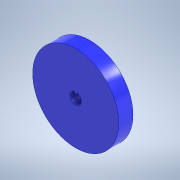
# Autodesk Inventor part: celestronMountDecHandle
Saved by Autodesk Inventor 2021.1 (Build 251245000, 245)
## iProperties
Created: 2020-07-29
Part Number: celestronMountDecHandle
Material: PC/ABS Plastic
Document SubType Name: Modeling
Designer: robst
Density: 0.357273 g/cm^3
Appearance: Blue - Wall Paint - Glossy
Author: robst
Autodesk Inventor part; units mm, degrees
ref_plane "YZ Plane" through (0, 0, 0) normal (1, 0, 0) x (0, 1, 0)
ref_plane "XY Plane" through (0, 0, 0) normal (0, 0, 1) x (1, 0, 0)
sketch "Sketch1" plane through (0, 0, 0) normal (0, 0, 1) x (1, 0, 0)
  circle A0 centre (0, 0) radius 38.1
  dimension "d0" = 76.2
  constraints: 1 centre point, 1 coincident
  measures "d0" diameter of A0
extrude "Extrusion1" add sketch "Sketch1" against normal blind 12.7
sketch "Sketch2" plane through (0, 0, -12.7) normal (0, 0, -1) x (-1, 0, 0)
  circle A0 centre (0, 0) radius 15.1765
  dimension "d3" = 30.353
  constraints: 1 centre point, 1 coincident
  measures "d3" diameter of A0
extrude "Extrusion2" add sketch "Sketch2" along normal blind 12.7
sketch "Sketch3" plane through (0, 0, 0) normal (0, 0, 1) x (1, 0, 0)
  arc A0 (-1.1906, 4.8732) -> (1.1906, 4.8732) centre (0, 0) ccw
  line L0 (-1.1906, 4.8732) -> (-1.1906, 3.4285)
  line L1 (-1.1906, 3.4285) -> (1.1906, 3.4285)
  line L2 (1.1906, 3.4285) -> (1.1906, 4.8732)
  circle A1 centre (0, 0) radius 15.1765 projected
  dimension "d6" = 10.033
  dimension "d7" = 2.3813
  dimension "d8" = 1.4446
  dimension "d15" = 10.16
  constraints: 6 end point, 2 point on circle, 2 vertical, 1 centre point, 1 coincident, 1 horizontal, 1 parallel
  measures "d6" diameter of A0
  measures "d7" distance of L0.end L1.end
  measures "d8" distance of L0.start L0.end
  measures "d15" radial gap between concentric circles of A0 A1
extrude "Extrusion3" cut sketch "Sketch3" against normal through all contours L0 L1 L2 A0
ref_plane "Work Plane2" through (0, -15.1765, 0) normal (0, 1, 0) x (-1, 0, 0)
sketch "Sketch4" plane through (0, -15.1765, 0) normal (0, 1, 0) x (-1, 0, 0)
  line L0 (-15.1765, -12.7) -> (-15.1765, -25.4) projected
  line L1 (15.1765, -12.7) -> (15.1765, -25.4) projected
  line L2 (-38.1, -12.7) -> (38.1, -12.7) projected
  line L3 (-15.1765, -25.4) -> (15.1765, -25.4) projected
  line L4 (0, -25.4) -> (0, -12.7) construction
  point P0 (0, 0)
  point P1 (0, -19.05)
  constraints: 3 midpoint, 2 end point
hole "Hole1" at (0, -15.1765, -19.05) direction (0, 1, 0) diameter 5.1054 depth 11.43 counterbore diameter 6.5278 counterbore depth 7.874 clearance for "Hex Machine Screw" size "#10" standard "Ansi Unified Screw Threads"
equation "\"d0\" = outerDiameter"
equation "\"d1\" = handleThickness"
equation "\"d3\" = shaftOutsideDiameter"
equation "\"d4\" = shaftLength"
equation "\"d6\" = shaftDiameter"
equation "\"d7\" = keyWidth"
equation "\"d8\" = keyDepth"
equation "\"outerDiameter\" = 76.2"
equation "\"handleThickness\" = 12.7"
equation "\"totalLength\" = 25.4"
equation "\"shaftDiameter\" = 10.033"
equation "\"keyWidth\" = 2.38125"
equation "\"keyDepth\" = 1.44462"
equation "\"shaftLength\" = totalLength - handleThickness"
equation "\"shaftOutsideDiameter\" = shaftDiameter + 2 * setScrewDepth"
equation "\"setScrewDepth\" = 10.16"
equation "\"setScrewWorkPlane\" = 0.5 * shaftOutsideDiameter"
equation "\"d16\" = -setScrewWorkPlane"
body "Solid1"
